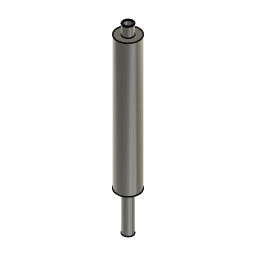
dribler (Autodesk Fusion 360 archive; units mm, degrees)
design "val"
Autodesk Fusion 360 part; units mm, degrees
sketch "Sketch1" plane through (0, 0, 0) normal (0, 0, 1) x (1, 0, 0)
  circle A0 centre (0, 0) radius 2
  circle A1 centre (0, 0) radius 4.5
  dimension "d1" = 4
  dimension "d2" = 9
  constraint coincident A0.centre A1.centre
  measures "d1" diameter of A0
  measures "d2" diameter of A1
extrude "Extrude1" add sketch "Sketch1" along normal blind 65 contours A0 | A1
extrude "Extrude2" cut sketch "Sketch1" along normal blind 10
extrude "Extrude3" add sketch "Sketch1" along normal blind 75 contours A0
sketch "Sketch2" plane through (0, 0, 75) normal (0, 0, 1) x (-1, 0, 0)
  circle A0 centre (0, 0) radius 2
  circle A1 centre (0, 0) radius 1.5
  dimension "d9" = 3
  constraint coincident A0.centre A1.centre
  measures "d9" diameter of A1
extrude "Extrude4" cut sketch "Sketch2" against normal blind 9 contours A1
extrude "Extrude5" cut 1 faces at (1.8203, -0.1739, 75) along direction (0, 0, -1) blind 6
extrude "Extrude6" add 1 faces at (0.637, 0.1965, 0) along direction (0, 0, -1) blind 6

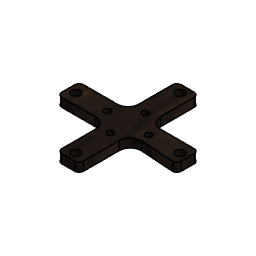
design "motor_holder"
Autodesk Fusion 360 part; units mm, degrees
sketch "Sketch1" plane through (0, 0, 0) normal (0, 0, 1) x (1, 0, 0)
  line L0 (0, 80) -> (0, -60) construction
  line L1 (-100, 0) -> (100, 0) construction
  circle A0 centre (0, 8) radius 1.5
  circle A1 centre (0, -8) radius 1.5
  line L2 (3, 27.5) -> (-3, 27.5)
  line L3 (-5, 25.5) -> (-5, 10)
  line L4 (-3, -27.5) -> (3, -27.5)
  line L5 (5, 10) -> (5, 25.5)
  line L6 (5, 27.5) -> (-5, -27.5) construction
  line L7 (-5, 27.5) -> (5, -27.5) construction
  line L8 (-10, -5) -> (-25.5, -5)
  line L9 (-27.5, -3) -> (-27.5, 3)
  line L10 (-25.5, 5) -> (-10, 5)
  line L11 (27.5, 3) -> (27.5, -3)
  line L12 (27.5, -5) -> (-27.5, 5) construction
  line L13 (-27.5, -5) -> (27.5, 5) construction
  arc A2 (-3, 27.5) -> (-5, 25.5) centre (-3, 25.5) ccw
  arc A3 (5, 25.5) -> (3, 27.5) centre (3, 25.5) ccw
  arc A4 (3, -27.5) -> (5, -25.5) centre (3, -25.5) ccw
  arc A5 (-5, -25.5) -> (-3, -27.5) centre (-3, -25.5) ccw
  arc A6 (-27.5, -3) -> (-25.5, -5) centre (-25.5, -3) ccw
  arc A7 (-25.5, 5) -> (-27.5, 3) centre (-25.5, 3) ccw
  arc A8 (27.5, 3) -> (25.5, 5) centre (25.5, 3) ccw
  arc A9 (25.5, -5) -> (27.5, -3) centre (25.5, -3) ccw
  arc A10 (-10, 5) -> (-5, 10) centre (-10, 10) ccw
  line L14 (-5, -25.5) -> (-5, -10)
  line L15 (25.5, 5) -> (10, 5)
  arc A11 (5, 10) -> (10, 5) centre (10, 10) ccw
  line L16 (5, -25.5) -> (5, -8.9884)
  arc A12 (-5, -10) -> (-10, -5) centre (-10, -10) ccw
  line L17 (10.3291, -3.9993) -> (25.5, -5)
  arc A13 (10.3291, -3.9993) -> (5, -8.9884) centre (10, -8.9884) ccw
  circle A14 centre (0, -24) radius 2
  circle A15 centre (24, 0) radius 2
  circle A16 centre (0, 24) radius 2
  circle A17 centre (-24, 0) radius 2
  circle A18 centre (-9.5, 0) radius 1.5
  circle A19 centre (9.5, 0) radius 1.5
  dimension "d1" = 3
  dimension "d2" = 8
  dimension "d4" = 360
  dimension "d5" = 10
  dimension "d6" = 55
  dimension "d7" = 55
  dimension "d8" = 10
  dimension "d9" = 2
  dimension "d10" = 2
  dimension "d11" = 5
  dimension "d12" = 5
  dimension "d13" = 5
  dimension "d14" = 5
  dimension "d15" = 4
  dimension "d16" = 24
  dimension "d18" = 360
  dimension "d21" = 3
  dimension "d22" = 9.5
  constraint vertical L0
  constraint horizontal L1
  constraint coincident L0 A0.centre
  constraint horizontal L2
  constraint perpendicular L2 L3
  constraint parallel L2 L4
  constraint parallel L3 L5
  constraint coincident L6 origin
  constraint coincident L7 origin
  constraint horizontal L8
  constraint perpendicular L8 L9
  constraint parallel L8 L10
  constraint parallel L9 L11
  constraint coincident L12 origin
  constraint coincident L13 origin
  constraint coincident L7.start L2
  constraint coincident L7.start L3
  constraint tangent L2 A2
  constraint tangent L3 A2
  constraint coincident L6.start L2
  constraint coincident L6.start L5
  constraint tangent L2 A3
  constraint tangent L5 A3
  constraint equal A2 A3
  constraint coincident L7.end L5
  constraint coincident L7.end L4
  constraint tangent L5 A4
  constraint tangent L4 A4
  constraint equal A2 A4
  constraint coincident L6.end L3
  constraint coincident L6.end L4
  constraint tangent L3 A5
  constraint tangent L4 A5
  constraint equal A2 A5
  constraint coincident L13.start L8
  constraint coincident L13.start L9
  constraint tangent L8 A6
  constraint tangent L9 A6
  constraint equal A2 A6
  constraint coincident L12.end L10
  constraint coincident L12.end L9
  constraint tangent L10 A7
  constraint tangent L9 A7
  constraint equal A2 A7
  constraint coincident L13.end L10
  constraint coincident L13.end L11
  constraint tangent L10 A8
  constraint tangent L11 A8
  constraint equal A2 A8
  constraint coincident L12.start L8
  constraint coincident L12.start L11
  constraint tangent L8 A9
  constraint tangent L11 A9
  constraint coincident L10 A8.end
  constraint coincident L3 A5.start
  constraint tangent L10 A10
  constraint tangent L3 A10
  constraint tangent A5 L14
  constraint tangent A8 L15
  constraint coincident L5 A4.end
  constraint tangent L5 A11
  constraint tangent L15 A11
  constraint tangent A4 L16
  constraint coincident L8 A9.start
  constraint tangent L8 A12
  constraint tangent L14 A12
  constraint tangent L16 A13
  constraint tangent L17 A13
  constraint coincident L0 A14.centre
  constraint coincident L1 A18.centre
  constraint symmetric L0 A18 A19
  measures "d1" diameter of A0
  measures "d2" distance of L1 A0.centre
  measures "d5" distance of L6.end L7.end
  measures "d6" distance of L7.start L6.end
  measures "d7" distance of L12.end L13.end
  measures "d8" distance of L13.start L12.end
  measures "d9" radius of A2
  measures "d10" radius of A9
  measures "d11" radius of A10
  measures "d12" radius of A11
  measures "d13" radius of A12
  measures "d14" radius of A13
  measures "d15" diameter of A14
  measures "d16" distance of origin A14.centre
  measures "d21" diameter of A18
  measures "d22" distance of origin A18.centre
extrude "Extrude1" add sketch "Sketch1" along normal blind 4
sketch "Sketch2" plane through (0, 0, 0) normal (0, 0, 1) x (1, 0, 0)
  circle A0 centre (0, -24) radius 2
  circle A1 centre (0, 24) radius 2
  circle A2 centre (0, 8) radius 1.5
  circle A3 centre (0, -8) radius 1.5
  circle A4 centre (24, 0) radius 2
  circle A5 centre (-24, 0) radius 2
  arc A6 (25.5, -5) -> (27.5, -3) centre (25.5, -3) ccw
  line L0 (27.5, -3) -> (27.5, 3)
  arc A7 (27.5, 3) -> (25.5, 5) centre (25.5, 3) ccw
  line L1 (25.5, 5) -> (10, 5)
  arc A8 (5, 10) -> (10, 5) centre (10, 10) ccw
  line L2 (5, 10) -> (5, 25.5)
  arc A9 (5, 25.5) -> (3, 27.5) centre (3, 25.5) ccw
  line L3 (3, 27.5) -> (-3, 27.5)
  arc A10 (-3, 27.5) -> (-5, 25.5) centre (-3, 25.5) ccw
  line L4 (-5, 25.5) -> (-5, 10)
  arc A11 (-10, 5) -> (-5, 10) centre (-10, 10) ccw
  line L5 (-10, 5) -> (-25.5, 5)
  arc A12 (-25.5, 5) -> (-27.5, 3) centre (-25.5, 3) ccw
  line L6 (-27.5, 3) -> (-27.5, -3)
  arc A13 (-27.5, -3) -> (-25.5, -5) centre (-25.5, -3) ccw
  line L7 (-25.5, -5) -> (-10, -5)
  arc A14 (-5, -10) -> (-10, -5) centre (-10, -10) ccw
  line L8 (-5, -10) -> (-5, -25.5)
  arc A15 (-5, -25.5) -> (-3, -27.5) centre (-3, -25.5) ccw
  line L9 (-3, -27.5) -> (3, -27.5)
  arc A16 (3, -27.5) -> (5, -25.5) centre (3, -25.5) ccw
  line L10 (5, -25.5) -> (5, -8.9884)
  arc A17 (10.3291, -3.9993) -> (5, -8.9884) centre (10, -8.9884) ccw
  line L11 (10.3291, -3.9993) -> (25.5, -5)
  circle A18 centre (-9.5, 0) radius 1.5
  circle A19 centre (9.5, 0) radius 1.5
equation "d2 = ( ( 13 + 3 ) / 2 ) * 1 mm"
equation "d22 = ( ( 16 + 3 ) / 2 ) * 1 mm"

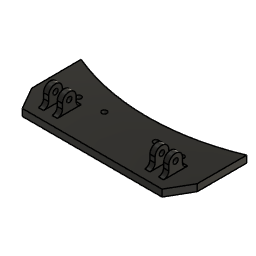
design "dribler_holder"
Autodesk Fusion 360 part; units mm, degrees
sketch "Sketch1" plane through (0, 0, 0) normal (0, 0, 1) x (1, 0, 0)
  line L0 (48.2374, 7.8721) -> (70.6242, 20.7971)
  line L1 (33.2374, -25.1279) -> (48.2374, 0.8529)
  circle A0 centre (-51.282, 21.1769) radius 1.5
  circle A1 centre (51.282, 21.1769) radius 1.5
  arc A2 (-55.6617, 33.0769) -> (-70.6242, 20.7971) centre (0, -50) ccw
  circle A3 centre (15, -20) radius 1.5
  line L2 (-33.2743, -25.1279) -> (33.2374, -25.1279)
  line L3 (-48.2374, 7.8721) -> (-48.2005, 0.8529)
  arc A4 (70.6242, 20.7971) -> (55.6617, 33.0769) centre (0, -50) ccw
  line L4 (-70.6242, 20.7971) -> (-48.2374, 7.8721)
  line L5 (-48.2005, 0.8529) -> (-33.2743, -25.1279)
  circle A5 centre (-15, -20) radius 1.5
  line L6 (48.2374, 0.8529) -> (48.2374, 7.8721)
  arc A6 (-55.6617, 33.0769) -> (55.6617, 33.0769) centre (0, 145) ccw
  line L7 (-40.7374, -12.1375) -> (40.7374, -12.1375)
  line L8 (48.2374, 7.8721) -> (48.2374, 29.6824)
  line L9 (-48.2374, 7.8721) -> (-48.3522, 29.7305)
  line L10 (0, -50) -> (0, 145) construction
  circle A7 centre (15, 10) radius 1.5
  circle A8 centre (30, 10) radius 1.5
  line L11 (126, 0) -> (-89, 0) construction
  line L12 (25, 5) -> (20, 5)
  line L13 (20, 5) -> (20, 15)
  line L14 (20, 15) -> (25, 15)
  line L15 (25, 15) -> (25, 5)
  line L16 (-25, 5) -> (-20, 5)
  line L17 (-20, 15) -> (-25, 15)
  line L18 (-25, 15) -> (-25, 5)
  line L19 (-20, 5) -> (-20, 15)
  circle A9 centre (-30, 10) radius 1.5
  circle A10 centre (-15, 10) radius 1.5
  line L20 (48.2374, 19.9303) -> (-48.3007, 19.9303)
  dimension "d57" = 3
  dimension "d58" = 3
  dimension "d59" = 10
  dimension "d60" = 10
  dimension "d61" = 5
  dimension "d62" = 20
  dimension "d63" = 5
  dimension "d64" = 5
  constraint midpoint L5 L7.start
  constraint midpoint L1 L7.end
  constraint parallel L2 L7
  constraint coincident A6 L8.end
  constraint perpendicular L7 L8
  constraint coincident A6 L9.end
  constraint parallel L3 L9
  constraint coincident A2.centre A4.centre
  constraint coincident A6.centre L10.end
  constraint vertical L10
  constraint horizontal L11
  constraint horizontal L12
  constraint vertical L13
  constraint horizontal L14
  constraint vertical L15
  constraint symmetric L10 A7 A10
  constraint symmetric L10 A8 A9
  constraint symmetric L10 L12.start L16.start
  constraint symmetric L10 L12.end L16.end
  constraint symmetric L10 L13.end L17.start
  constraint symmetric L10 L14.end L17.end
  constraint coincident L8 L20.start
  constraint coincident L9 L20.end
  constraint perpendicular L8 L20
  measures "d57" diameter of A7
  measures "d58" diameter of A8
  measures "d59" distance of A8.centre L11
  measures "d60" distance of A7.centre L11
  measures "d61" distance of L11 L12
  measures "d62" distance of L10 L13
  measures "d63" distance of A8.centre L15
  measures "d64" distance of A7.centre L13
extrude "Extrude7" add sketch "Sketch1" along normal blind 4 contours L1 L3 L5 L6 L7 L8 L9 L20 | A6 L8 L9 L20 | L12 L13 L14 L15 | L16 L17 L18 L19
extrude "Extrude8" add sketch "Sketch1" against normal blind 6 contours L12 L13 L14 L15 | L16 L17 L18 L19
sketch "Sketch5" plane through (0, 0, 4) normal (0, 0, 1) x (-1, 0, 0)
  circle A0 centre (30, -10) radius 1.5
  circle A1 centre (15, -10) radius 1.5
  circle A2 centre (-30, -10) radius 1.5
  circle A3 centre (-15, -10) radius 1.5
  line L0 (48.2005, -0.8529) -> (40.7374, 12.1375)
  line L1 (40.7374, 12.1375) -> (-40.7374, 12.1375)
  line L2 (-40.7374, 12.1375) -> (-48.2374, -0.8529)
  line L3 (-48.2374, -0.8529) -> (-48.2374, -29.6824)
  arc A4 (48.3522, -29.7305) -> (-48.2374, -29.6824) centre (0, -145) ccw
  line L4 (48.3522, -29.7305) -> (48.2005, -0.8529)
  line L5 (0, 35) -> (0, -35) construction
  line L6 (-36.5, 4) -> (-24.5, 4)
  line L7 (-24.5, 4) -> (-24.5, -4)
  line L8 (-24.5, -4) -> (-36.5, -4)
  line L9 (-36.5, -4) -> (-36.5, 4)
  line L10 (-36.5, 4) -> (-32.5, 4)
  line L11 (-32.5, 4) -> (-32.5, -4)
  line L12 (-32.5, -4) -> (-36.5, -4)
  line L13 (-36.5, -4) -> (-36.5, 4)
  line L14 (-24.5, 4) -> (-28.5, 4)
  line L15 (-28.5, 4) -> (-28.5, -4)
  line L16 (-28.5, -4) -> (-24.5, -4)
  line L17 (-24.5, -4) -> (-24.5, 4)
  line L18 (-100, 0) -> (80, 0) construction
  line L19 (24.5, 4) -> (24.5, -4)
  line L20 (28.5, -4) -> (24.5, -4)
  line L21 (24.5, -4) -> (36.5, -4)
  line L22 (36.5, 4) -> (32.5, 4)
  line L23 (36.5, -4) -> (36.5, 4)
  line L24 (36.5, -4) -> (36.5, 4)
  line L25 (32.5, -4) -> (36.5, -4)
  line L26 (32.5, 4) -> (32.5, -4)
  line L27 (28.5, 4) -> (28.5, -4)
  line L28 (24.5, 4) -> (28.5, 4)
  line L29 (36.5, 4) -> (24.5, 4)
  line L30 (24.5, -4) -> (24.5, 4)
  dimension "d69" = 12
  dimension "d70" = 8
  dimension "d71" = 4
  dimension "d72" = 8
  dimension "d73" = 4
  dimension "d74" = 8
  dimension "d75" = 32.5
  dimension "d76" = 4
  constraint vertical L5
  constraint horizontal L6
  constraint vertical L7
  constraint horizontal L8
  constraint vertical L9
  constraint horizontal L10
  constraint vertical L11
  constraint horizontal L12
  constraint vertical L13
  constraint horizontal L14
  constraint vertical L15
  constraint horizontal L16
  constraint vertical L17
  constraint perpendicular L13 L18
  constraint symmetric L5 L6.start L22.start
  constraint symmetric L5 L6.end L19.start
  constraint symmetric L5 L7.end L19.end
  constraint symmetric L5 L8.end L21.end
  constraint symmetric L5 L10.end L22.end
  constraint symmetric L5 L11.end L25.start
  constraint symmetric L5 L14.end L27.start
  constraint symmetric L5 L15.end L20.start
  measures "d69" distance of L6.start L6.end
  measures "d70" distance of L6.start L8.end
  measures "d71" distance of L6.start L10.end
  measures "d72" distance of L6.start L8.end
  measures "d73" distance of L6.end L14.end
  measures "d74" distance of L6.end L7.end
  measures "d75" distance of L5 L11
  measures "d76" distance of L6 L18
extrude "Extrude9" add sketch "Sketch5" along normal blind 10 contours L6 L8 L9 L10 L11 L12 L13 | L6 L7 L8 L14 L15 L16 L17 | L19 L20 L21 L27 L28 L29 L30 | L21 L22 L23 L24 L25 L26 L29
sketch "Sketch6" plane through (36.5, 0, 0) normal (1, 0, 0) x (0, 1, 0)
  line L0 (-4, 4) -> (4, 4)
  line L1 (4, 4) -> (4, 14)
  line L2 (4, 14) -> (-4, 14)
  line L3 (-4, 14) -> (-4, 4)
  line L4 (-4, 14) -> (4, 14)
  line L5 (4, 14) -> (4, 4)
  line L6 (4, 4) -> (-4, 4)
  line L7 (-4, 4) -> (-4, 14)
  circle A0 centre (0, 10) radius 1.5
  dimension "d79" = 3
  dimension "d80" = 4
  dimension "d81" = 4
  constraint horizontal L4
  constraint vertical L5
  constraint horizontal L6
  constraint vertical L7
  constraint coincident L0.end L1.start
  constraint coincident L2.end L3.start
  measures "d79" diameter of A0
  measures "d80" distance of L4 A0.centre
  measures "d81" distance of L5 A0.centre
extrude "Extrude10" cut sketch "Sketch6" against normal blind 170 contours A0
fillet "Fillet1" radius 4 8 edges at (34.5, -4, 14) (34.5, 4, 14) (26.5, -4, 14) (26.5, 4, 14) (-26.5, -4, 14) (-26.5, 4, 14) (-34.5, -4, 14) (-34.5, 4, 14)
fillet "Fillet2" radius 3 8 edges at (26.5, 4, 4) (34.5, 4, 4) (26.5, -4, 4) (34.5, -4, 4) (-34.5, -4, 4) (-26.5, -4, 4) (-34.5, 4, 4) (-26.5, 4, 4)
extrude "Extrude11" cut 1 faces at (-32.5, -0.0374, 6.6706) along direction (-1, 0, 0) blind 1
extrude "Extrude12" cut 1 faces at (32.5, 0.0374, 6.6706) along direction (1, 0, 0) blind 1
extrude "Extrude13" cut 1 faces at (-24.5, 0.0374, 6.6706) along direction (-1, 0, 0) blind 1
extrude "Extrude14" cut 1 faces at (24.5, 0.0374, 6.6706) along direction (1, 0, 0) blind 1
equation "d75 = ( 65 / 2 ) * 1 mm"

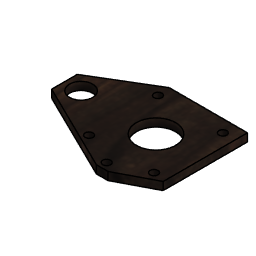
design "dribler_polovinka"
Autodesk Fusion 360 part; units mm, degrees
sketch "Sketch1" plane through (0, 0, 0) normal (0, 0, 1) x (1, 0, 0)
  line L0 (-119.7889, 0) -> (120, 0) construction
  line L1 (0, 100) -> (0, -100) construction
  circle A0 centre (0, 0) radius 10
  circle A1 centre (0, -25) radius 2
  circle A2 centre (-38, 0) radius 5.875
  circle A3 centre (-16.4591, -17.4671) radius 2
  circle A4 centre (-16.4591, 17.4671) radius 2
  circle A5 centre (16.4591, -17.4671) radius 2
  circle A6 centre (16.4591, 17.4671) radius 2
  line L2 (-16.4591, 17.4671) -> (16.4591, -17.4671) construction
  line L3 (16.4591, 17.4671) -> (-16.4591, -17.4671) construction
  line L4 (-16.4591, 17.4671) -> (-16.4591, -17.4671) construction
  line L5 (16.4591, -17.4671) -> (-16.4591, -17.4671) construction
  line L6 (16.4591, 17.4671) -> (16.4591, -17.4671) construction
  line L7 (16.4591, 17.4671) -> (-16.4591, 17.4671) construction
  line L8 (-46.1604, 6.2301) -> (-46.1604, -6.7642)
  line L9 (-46.1604, -6.7642) -> (-1.6176, -28.6203)
  line L10 (-1.6176, -28.6203) -> (4.2426, -28.6203)
  line L11 (4.2426, -28.6203) -> (22.669, -19.0288)
  line L12 (22.669, -19.0288) -> (22.669, 23.7134)
  line L13 (22.669, 23.7134) -> (-17.0215, 23.7134)
  line L14 (-17.0215, 23.7134) -> (-46.1604, 6.2301)
  point P0 (19.151, -29.5459)
  point P1 (-43.849, -29.5459)
  point P2 (-53.4128, 17.4541)
  point P3 (19.151, 17.4541)
  dimension "d21" = 20
  dimension "d22" = 4
  dimension "d23" = 25
  dimension "d26" = 11.75
  dimension "d27" = 38
  dimension "d44" = 48
  constraint horizontal L0
  constraint vertical L1
  constraint coincident A0.centre origin
  constraint coincident L1 A1.centre
  constraint coincident L0 A2.centre
  constraint coincident A4.centre L2.start
  constraint coincident A5.centre L2.end
  constraint coincident A6.centre L3.start
  constraint coincident A3.centre L3.end
  constraint vertical L4
  constraint perpendicular L4 L5
  constraint perpendicular L5 L6
  constraint perpendicular L4 L7
  constraint midpoint L2 A0.centre
  constraint perpendicular L0 L8
  constraint perpendicular L1 L10
  constraint perpendicular L0 L12
  constraint perpendicular L12 L13
  measures "d21" diameter of A0
  measures "d22" diameter of A1
  measures "d23" distance of A0.centre A1.centre
  measures "d26" diameter of A2
  measures "d27" distance of A0.centre A2.centre
  measures "d44" distance of A6.centre A3.centre
extrude "Extrude1" add sketch "Sketch1" along normal blind 4
sketch "Sketch2" plane through (0, 0, 4) normal (0, 0, 1) x (-1, 0, 0)
  circle A0 centre (0, 0) radius 10
  circle A1 centre (38, 0) radius 5.875
  circle A2 centre (0, 25) radius 2
  line L0 (17.0215, -23.7134) -> (46.1604, -6.2301)
  line L1 (46.1604, -6.2301) -> (46.1604, 6.7642)
  line L2 (46.1604, 6.7642) -> (1.6176, 28.6203)
  line L3 (1.6176, 28.6203) -> (-4.2426, 28.6203)
  line L4 (-4.2426, 28.6203) -> (-22.669, 19.0288)
  line L5 (-22.669, 19.0288) -> (-22.669, -23.7134)
  line L6 (-22.669, -23.7134) -> (17.0215, -23.7134)
  circle A3 centre (16.4591, -17.4671) radius 2
  circle A4 centre (-16.4591, 17.4671) radius 2
  circle A5 centre (16.4591, 17.4671) radius 2
  circle A6 centre (-16.4591, -17.4671) radius 2

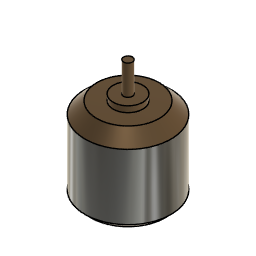
design "motor_1000KV"
Autodesk Fusion 360 part; units mm, degrees
sketch "Sketch1" plane through (0, 0, 0) normal (0, 0, 1) x (1, 0, 0)
  circle A0 centre (0, 0) radius 14.5
  line L0 (0, 30) -> (0, -25) construction
  line L1 (-30, 0) -> (26, 0) construction
  circle A1 centre (0, -10) radius 1.5
  circle A2 centre (10, 0) radius 1.5
  circle A3 centre (0, 10) radius 1.5
  circle A4 centre (-10, 0) radius 1.5
  dimension "d1" = 29
  dimension "d3" = 3
  dimension "d4" = 10
  dimension "d6" = 360
  constraint coincident A0.centre origin
  constraint vertical L0
  constraint horizontal L1
  constraint coincident L0 A1.centre
  measures "d1" diameter of A0
  measures "d3" diameter of A1
  measures "d4" distance of L1 A1.centre
extrude "Extrude1" add sketch "Sketch1" along normal blind 30
extrude "Extrude2" add sketch "Sketch1" along normal blind 30 contours A1 | A2 | A3 | A4
extrude "Extrude3" cut sketch "Sketch1" along normal blind 10 contours A1 | A2 | A3 | A4
sketch "Sketch2" plane through (0, 0, 30) normal (0, 0, 1) x (-1, 0, 0)
  circle A0 centre (0, 0) radius 14.5
  circle A1 centre (0, 0) radius 1.5
  dimension "d13" = 3
  constraint concentric A0 A1
  measures "d13" diameter of A1
extrude "Extrude4" add sketch "Sketch2" along normal blind 10 contours A1
extrude "Extrude5" cut 1 faces at (10.1127, -0.7204, 30) along direction (0, 0, -1) blind 2
sketch "Sketch3" plane through (0, 0, 28) normal (0, 0, 1) x (-1, 0, 0)
  circle A0 centre (0, 0) radius 1.5
  circle A1 centre (0, 0) radius 14.5
  circle A2 centre (0, 0) radius 5
  dimension "d18" = 10
  constraint coincident A0.centre A1.centre
  measures "d18" diameter of A2
extrude "Extrude6" add sketch "Sketch3" along normal blind 2 contours A2
chamfer "Chamfer1" distance 4 angle 45 1 edges at (-13.5187, 5.2434, 28)
chamfer "Chamfer2" distance 2 angle 45 1 edges at (-13.5187, -5.2434, 0)
